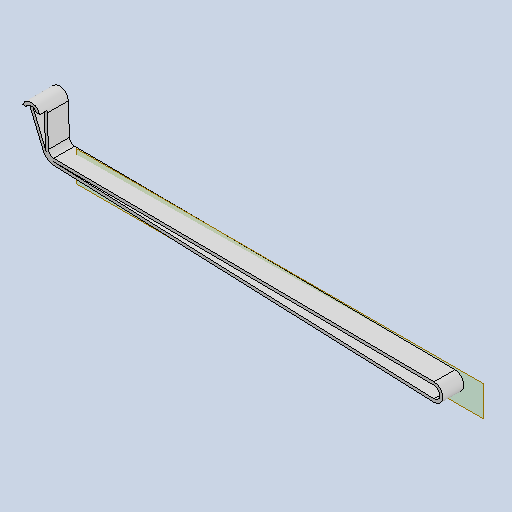
# Autodesk Inventor part: Cata rubber bands
Saved by Autodesk Inventor 2023.2 (Build 272271030, 271C)
## iProperties
Created: 2023-05-20
Part Number: Cata rubber bands
Material: Generic
Document SubType Name: Modeling
Designer: Main Account
Density: 1 g/cm^3
Appearance: Default
Author: Main Account
Autodesk Inventor part; units mm, degrees
ref_plane "YZ Plane" through (0, 0, 0) normal (1, 0, 0) x (0, 1, 0)
ref_plane "XZ Plane" through (0, 0, 0) normal (0, 1, 0) x (-1, 0, 0)
ref_plane "XY Plane" through (0, 0, 0) normal (0, 0, 1) x (1, 0, 0)
sketch "Sketch1" plane through (0, 0, 0) normal (0, 0, 1) x (1, 0, 0)
  circle A0 centre (-218.2217, -192.1682) radius 3.0353 construction
  circle A1 centre (-209.2225, -209.7173) radius 3.0353 construction
  circle A2 centre (15.875, -215.9) radius 3.0353 construction
  arc A3 (-212.2548, -209.8537) -> (-209.1953, -212.7525) centre (-209.2225, -209.7173) ccw
  arc A4 (-214.8089, -192.0147) -> (-221.3625, -193.5122) centre (-218.2217, -192.1682) ccw
  arc A5 (-213.0607, -191.936) -> (-222.9714, -194.2008) centre (-218.2217, -192.1682) ccw
  arc A6 (15.802, -219.3155) -> (15.8444, -212.4838) centre (15.875, -215.9) ccw
  arc A7 (15.7646, -221.0651) -> (15.8287, -210.7339) centre (15.875, -215.9) ccw
  line L0 (-212.2548, -209.8537) -> (-213.0607, -191.936)
  line L1 (-215.2308, -212.2885) -> (-222.9714, -194.2008)
  line L2 (-221.3625, -193.5122) -> (-213.6219, -211.6)
  line L3 (-214.003, -209.9323) -> (-214.8089, -192.0147)
  line L4 (-209.1953, -212.7525) -> (15.8287, -210.7339)
  line L5 (15.8444, -212.4838) -> (-209.1796, -214.5024)
  line L6 (15.802, -219.3155) -> (-209.3248, -214.5015)
  line L7 (-209.3623, -216.2511) -> (15.7646, -221.0651)
  arc A8 (-214.003, -209.9323) -> (-209.1796, -214.5024) centre (-209.2225, -209.7173) ccw
  arc A9 (-215.2308, -212.2885) -> (-209.3623, -216.2511) centre (-209.2225, -209.7173) ccw
  arc A10 (-204.6436, -214.6016) -> (-204.4975, -214.4604) centre (-209.2225, -209.7173) ccw
  point P0 (0, 0)
  point P1 (-192.7723, -212.6051)
  point P2 (-183.4432, -220.9999)
  point P3 (-202.7453, -212.6946)
  point P4 (-199.5727, -216.4604)
  point P5 (-186.4, -216.7421)
  dimension "d0" = 0
  dimension "d2" = 0.381
  dimension "d3" = 1.75
  dimension "d9" = 1.75
  dimension "d10" = 1.75
  dimension "d11" = 0.381
  dimension "d12" = 1.75
  constraints: 18 point on circle, 16 end point, 16 tangent, 8 centre point, 2 point on line
  measures "d0" radial gap between concentric circles of A1 A3
  measures "d2" radial gap between concentric circles of A0 A4
  measures "d3" radial gap between concentric circles of A4 A5
  measures "d9" radial gap between concentric circles of A3 A8
  measures "d10" radial gap between concentric circles of A9 A8
  measures "d11" radial gap between concentric circles of A6 A2
  measures "d12" radial gap between concentric circles of A7 A6
extrude "main bands" add sketch "Sketch1" along normal blind 12.7 and the other way blind 3.81
sketch "Sketch2" plane through (15.7646, -221.0651, -3.81) normal (-0.0213787, -0.9997714, 0) x (0.9997714, -0.0213787, 0)
  line L0 (5.1663, 0) -> (5.1663, 16.51) projected
  line L1 (-225.1783, 16.51) -> (0, 16.51) projected
  line L2 (0, 0) -> (-225.1783, 0) projected
  line L3 (-239.7169, 0) -> (-239.7169, 16.51) projected
  line L4 (-239.7169, 0) -> (-229.3956, 0) projected
  line L5 (5.1663, 4.318) -> (-239.7169, 0)
  line L6 (0, 0) -> (5.1663, 0)
  line L7 (-239.7169, 0) -> (-225.1783, 0)
  line L8 (-229.3956, 16.51) -> (-239.7169, 16.51) projected
  line L9 (-239.7169, 16.51) -> (-225.1783, 16.51)
  line L10 (5.1663, 16.51) -> (0, 16.51)
  line L11 (5.1663, 16.51) -> (-239.7169, 12.192)
  point P0 (-20.487, 3.81)
  point P1 (-239.2557, 0)
  point P2 (-239.2557, 16.51)
  dimension "d17" = 4.318
  dimension "d18" = 4.318
  constraints: 12 end point, 2 horizontal, 2 point on line, 1 collinear, 1 parallel
  measures "d17" distance of L0.start L5.start
  measures "d18" distance of L3.end L11.end
extrude "diagonal cuts" cut sketch "Sketch2" against normal blind 25.4 contours L6 L2 L7 L4 L5 L0 | L11 L3 L8 L9 L1 L10
ref_plane "inside edge" through (0, 0, 0) normal (0, 0, -1) x (-1, 0, 0)
body "Solid1"
